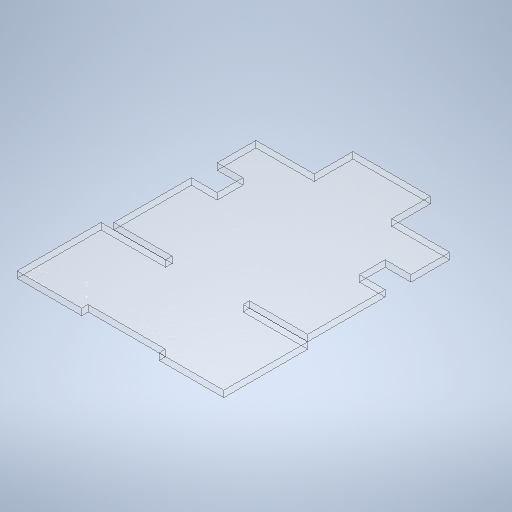
# Autodesk Inventor part: HOOD_1
Saved by Autodesk Inventor 2025.3 (Build 293356030, 356C)
## iProperties
Created: 2026-06-30
Part Number: HOOD_1
Material: Acrylic
Document SubType Name: Modeling
Designer: user
Density: 1.188 g/cm^3
Appearance: Transparent - Clear
Author: user
Autodesk Inventor part; units mm, degrees
ref_plane "YZ Plane" through (0, 0, 0) normal (1, 0, 0) x (0, 1, 0)
ref_plane "XZ Plane" through (0, 0, 0) normal (0, 1, 0) x (-1, 0, 0)
ref_plane "XY Plane" through (0, 0, 0) normal (0, 0, 1) x (1, 0, 0)
sketch "Sketch1" plane through (0, 0, 0) normal (0, 1, 0) x (-1, 0, 0)
  line L0 (155, -70) -> (155, -210)
  line L1 (155, -210) -> (5, -210)
  line L2 (5, -210) -> (5, -70)
  line L3 (50, -210) -> (110, -210)
  line L4 (5, -70) -> (155, -70)
  line L5 (5, -70) -> (55, -70)
  line L6 (155, -150) -> (135, -150)
  line L7 (135, -150) -> (135, -130)
  line L8 (135, -130) -> (155, -130)
  line L9 (155, -130) -> (155, -150)
  line L10 (5, -150) -> (25, -150)
  line L11 (25, -150) -> (25, -130)
  line L12 (25, -130) -> (5, -130)
  line L13 (5, -180) -> (155, -180) construction
  line L14 (50, -180) -> (110, -180)
  line L15 (110, -180) -> (110, -210)
  line L16 (110, -210) -> (50, -210)
  line L17 (50, -210) -> (50, -180)
  line L18 (110, -210) -> (50, -210)
  line L19 (155, -180) -> (110, -180)
  line L20 (50, -180) -> (5, -180)
  line L21 (135, -30) -> (155, -30)
  line L22 (160, -70) -> (0, -70)
  line L23 (0, -70) -> (0, 0)
  line L24 (0, 0) -> (160, 0)
  line L25 (160, 0) -> (160, -70)
  line L26 (80, -210) -> (80, 0) construction
  line L27 (0, -70) -> (50, -70)
  line L28 (50, -70) -> (50, -65)
  line L29 (50, -65) -> (0, -65)
  line L30 (0, -65) -> (0, -70)
  line L31 (155, -70) -> (105, -70)
  line L32 (160, -70) -> (110, -70)
  line L33 (110, -70) -> (110, -65)
  line L34 (110, -65) -> (160, -65)
  line L35 (160, -65) -> (160, -70)
  line L36 (110, 0) -> (50, 0)
  line L37 (50, 0) -> (50, -5)
  line L38 (50, -5) -> (110, -5)
  line L39 (110, -5) -> (110, 0)
  point P0 (5, -100)
  point P1 (5, -120)
  point P2 (160, -65)
  point P3 (155, 0)
  point P4 (135, 0)
  point P5 (0, -65)
  point P6 (50, -70)
  point P7 (110, -70)
  point P8 (50, 0)
  point P9 (50, -70)
  point P10 (110, -70)
  point P11 (155, -70)
  point P12 (5, -70)
  dimension "d10" = 20
  dimension "d11" = 20
  dimension "d18" = 150
  dimension "d19" = 160
  dimension "d20" = 80
  dimension "d21" = 45
  dimension "d22" = 45
  dimension "d23" = 50
  dimension "d24" = 5
  dimension "d25" = 5
  dimension "d26" = 30
  dimension "d27" = 110
  dimension "d28" = 70
  dimension "d29" = 210
  dimension "d30" = 20
  constraints: 80 end point, 12 parallel, 10 point on line, 9 perpendicular, 8 horizontal, 4 symmetric about line, 3 collinear, 2 midpoint, 1 coincident
  measures "d10" distance of L7.end L8.end
  measures "d11" distance of L6.end L7.end
  measures "d18" distance of L13.start L13.end
  measures "d19" distance of L23.end L24.end
  measures "d20" distance between parallel lines of L23 L26
  measures "d21" distance between parallel lines of L2 L17
  measures "d22" distance between parallel lines of L0 L15
  measures "d23" distance of L29.end L28.end
  measures "d24" distance of L28.end L27.end
  measures "d25" distance of L37.end L36.end
  measures "d26" distance between parallel lines of L1 L13
  measures "d27" distance between parallel lines of L22 L13
  measures "d28" distance between parallel lines of L24 L4
  measures "d29" distance between parallel lines of L24 L1
  measures "d30" distance of L10.start L10.end
extrude "Extrusion1" add sketch "Sketch1" along normal blind 5 contours L0 L8 L7 L6 L19 L14 L20 L2 L10 L11 L12 L4 | L4 L28 L29 L23 L24 L37 L38 L39 L25 L34 L33 | L15 L1 L17 L14
body "Solid1"
